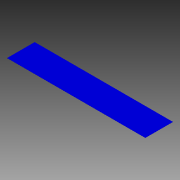
# Autodesk Inventor part: wall
Saved by Autodesk Inventor 2014 (Build 180170000, 170)
## iProperties
Created: 2015-04-22
Part Number: wall
Material: Generic
Document SubType Name: Modeling
Designer: Vladyslav
Density: 1 g/cm^3
Appearance: Default
Author: Vladyslav
Autodesk Inventor part; units mm, degrees
ref_plane "YZ Plane" through (0, 0, 0) normal (1, 0, 0) x (0, 1, 0)
ref_plane "XZ Plane" through (0, 0, 0) normal (0, 1, 0) x (-1, 0, 0)
ref_plane "XY Plane" through (0, 0, 0) normal (0, 0, 1) x (1, 0, 0)
sketch "Sketch2" plane through (0, 0, 0) normal (0, 0, 1) x (1, 0, 0)
  line L0 (0, 0) -> (100000, 0)
  line L1 (100000, 0) -> (100000, 20000)
  line L2 (100000, 20000) -> (0, 20000)
  line L3 (0, 20000) -> (0, 0)
  dimension "d0" = 100000
  dimension "d1" = 20000
  constraints: 8 end point, 2 parallel, 1 horizontal, 1 perpendicular
  measures "d0" distance of L2.end L1.end
  measures "d1" distance of L1.end L0.end
extrude "Extrusion1" add sketch "Sketch2" along normal blind 40
body "Solid1"
